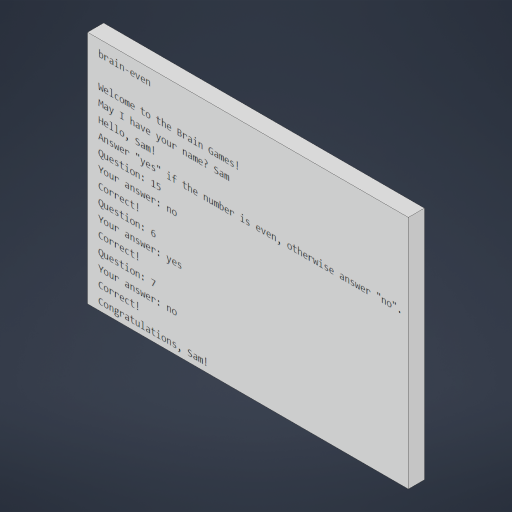
# Autodesk Inventor part: memo
Saved by Autodesk Inventor 2023.3 (Build 273359000, 359)
## iProperties
Created: 2024-01-15
Part Number: memo
Material: Типовые
Document SubType Name: Modeling
Designer: desig
Density: 1 g/cm^3
Appearance: По умолчанию
Author: desig
Autodesk Inventor part; units mm, degrees
ref_plane "YZ Plane" through (0, 0, 0) normal (1, 0, 0) x (0, 1, 0)
ref_plane "XZ Plane" through (0, 0, 0) normal (0, 1, 0) x (-1, 0, 0)
ref_plane "XY Plane" through (0, 0, 0) normal (0, 0, 1) x (1, 0, 0)
sketch "Эскиз1" plane through (0, 0, 0) normal (0, 0, 1) x (1, 0, 0)
  line L0 (0, 146.6893) -> (200, 146.6893)
  line L1 (200, 146.6893) -> (200, 0)
  line L2 (200, 0) -> (0, 0)
  line L3 (0, 0) -> (0, 146.6893)
  dimension "d1" = 200
  constraints: 1 coincident, 2 other
  measures "d1" distance of L0.start L0.end
extrude "Выдавливание1" add sketch "Эскиз1" against normal blind 10
decal "Декаль1"
